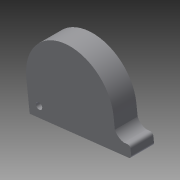
# Autodesk Inventor part: Surface Switch Trigger (High Hat)
Saved by Autodesk Inventor 2015 (Build 190159000, 159)
## iProperties
Created: 2015-02-05
Part Number: Surface Switch Trigger (High Hat)
Material: Generic
Document SubType Name: Modeling
Designer: robotics
Density: 1 g/cm^3
Appearance: Default
Author: robotics
Autodesk Inventor part; units mm, degrees
ref_plane "YZ Plane" through (0, 0, 0) normal (1, 0, 0) x (0, 1, 0)
ref_plane "XZ Plane" through (0, 0, 0) normal (0, 1, 0) x (-1, 0, 0)
ref_plane "XY Plane" through (0, 0, 0) normal (0, 0, 1) x (1, 0, 0)
sketch "Sketch1" plane through (0, 0, 0) normal (0, 0, 1) x (1, 0, 0)
  line L0 (-14.534, 1.5317) -> (13.0836, 4.6943)
  arc A0 (8.8744, 12.5875) -> (-15.4807, 9.7985) centre (-3.3032, 11.193) ccw
  circle A1 centre (-11.9285, 4.7064) radius 0.889
  line L1 (11.7169, 7.6855) -> (12.7278, 7.8013)
  line L2 (13.7819, 5.5732) -> (13.6067, 7.103)
  arc A2 (9.2226, 9.5467) -> (11.7169, 7.6855) centre (12.1248, 10.8342) ccw
  arc A3 (13.6067, 7.103) -> (12.7278, 7.8013) centre (12.8181, 7.0127) ccw
  arc A4 (13.0836, 4.6943) -> (13.7819, 5.5732) centre (12.9933, 5.4829) ccw
  line L3 (-24.0434, 21.1552) -> (25.4307, 26.8206) construction
  line L4 (-25.7025, 27.3567) -> (12.868, 31.7735) construction
  line L5 (-14.534, 1.5317) -> (-15.4807, 9.7985)
  line L6 (9.821, 4.3207) -> (8.8744, 12.5875) construction
  line L7 (-24.6974, 8.7431) -> (27.8347, 14.7587) construction
  line L8 (-2.3565, 2.9262) -> (-5.4201, 29.6793) construction
  line L9 (8.8744, 12.5875) -> (9.2226, 9.5467)
  dimension "nail" = 1.778
  dimension "d37" = 3.175
  dimension "d38" = 0.7937
  dimension "d60" = 1.0109
  dimension "d61" = 3.1273
  dimension "d62" = 27.7981
  dimension "airspace" = 6.35
  dimension "d64" = 8.3208
  dimension "d65" = 12.2571
  constraints: 20 end point, 10 point on circle, 8 point on line, 6 tangent, 5 centre point, 4 perpendicular, 3 parallel, 1 collinear, 1 equal radius, 3 other
  measures "nail" diameter of A1
  measures "d37" radius of A2
  measures "d38" radius of A3
  measures "d60" horizontal distance of L1.start L1.end
  measures "d61" distance between parallel lines of L0 L1
  measures "d62" distance of L0.start L0.end
  measures "airspace" distance between parallel lines of L4 L3
  measures "d64" distance between parallel lines of L0 L7
  measures "d65" distance between parallel lines of L5 L8
extrude "Extrusion6" add sketch "Sketch1" along normal blind 6.35
body "Solid3"
